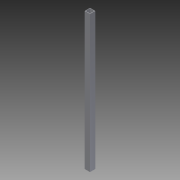
# Autodesk Inventor part: Tower Corner Mount
Saved by Autodesk Inventor 2013 (Build 170138000, 138)
## iProperties
Created: 2013-01-21
Part Number: Tower Corner Mount
Material: Aluminum 6061
Document SubType Name: Modeling
Designer: actoennies
Density: 2.71 g/cm^3
Mass: 274.52 g
Surface Area: 1279.23 cm^2
Volume: 101.299 cm^3
Author: actoennies
Autodesk Inventor part; units mm, degrees
ref_plane "YZ Plane" through (0, 0, 0) normal (1, 0, 0) x (0, 1, 0)
ref_plane "XZ Plane" through (0, 0, 0) normal (0, 1, 0) x (-1, 0, 0)
ref_plane "XY Plane" through (0, 0, 0) normal (0, 0, 1) x (1, 0, 0)
sketch "Sketch1" plane through (0, 0, 0) normal (0, 1, 0) x (-1, 0, 0)
  line L0 (0, 0) -> (-25.4, 0)
  line L1 (-25.4, 0) -> (-25.4, 25.4)
  line L2 (-25.4, 25.4) -> (0, 25.4)
  line L3 (0, 25.4) -> (0, 0)
  line L4 (-1.5875, 23.8125) -> (-23.8125, 23.8125)
  line L5 (-23.8125, 23.8125) -> (-23.8125, 1.5875)
  line L6 (-23.8125, 1.5875) -> (-1.5875, 1.5875)
  line L7 (-1.5875, 1.5875) -> (-1.5875, 23.8125)
  dimension "d0" = 25.4
  dimension "d2" = 25.4
  dimension "d3" = 1.5875
  constraints: 16 end point, 4 parallel, 2 perpendicular, 1 horizontal, 3 other
  measures "d0" distance of L1.end L2.end
  measures "d2" distance of L2.end L0.start
  measures "d3" distance between parallel lines of L2 L4
extrude "Extrusion1" add sketch "Sketch1" along normal blind 669.925
body "Solid1"
